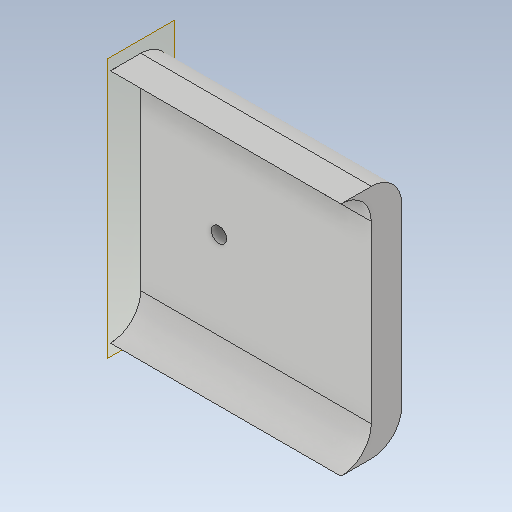
# Autodesk Inventor part: AzureKinectCradle
Saved by Autodesk Inventor 2020.2 (Build 242310000, 310)
## iProperties
Created: 2020-02-21
Part Number: AzureKinectCradle
Material: 一般
Document SubType Name: Modeling
Designer: gisen
Density: 1 g/cm^3
Appearance: 既定
Author: gisen
Autodesk Inventor part; units mm, degrees
ref_plane "YZ Plane" through (0, 0, 0) normal (1, 0, 0) x (0, 1, 0)
ref_plane "XZ Plane" through (0, 0, 0) normal (0, 1, 0) x (-1, 0, 0)
ref_plane "XY Plane" through (0, 0, 0) normal (0, 0, 1) x (1, 0, 0)
ref_plane "作業平面1" through (-27.3255, 41.0319, 38.0074) normal (1, 0, 0) x (0, 1, 0)
sketch "スケッチ2" plane through (-27.3255, 41.0319, 38.0074) normal (1, 0, 0) x (0, 1, 0)
  arc A0 (-51.6, -13.3) -> (-38.35, -26.55) centre (-38.35, -13.3) ccw
  line L0 (-51.6, 0) -> (-51.6, -13.3)
  arc A1 (-51.6, 0) -> (-38.35, -13.25) centre (-38.35, 0) ccw
  line L1 (38.35, -13.25) -> (-38.35, -13.25)
  arc A2 (38.35, -13.25) -> (51.6, 0) centre (38.35, 0) ccw
  line L2 (51.6, -13.3) -> (51.6, 0)
  arc A3 (38.35, -26.55) -> (51.6, -13.3) centre (38.35, -13.3) ccw
  line L3 (-38.35, -26.55) -> (38.35, -26.55)
  point P0 (-41.0319, -38.0074)
  constraints: 8 end point, 8 point on circle, 4 centre point
extrude "押し出し1" add sketch "スケッチ2" along normal blind 100.9
sketch "スケッチ3" plane through (-27.3255, 2.6819, 11.4574) normal (0, 0, -1) x (-1, 0, 0)
  line L0 (0, 76.7) -> (-100.9, 76.7) projected
  line L1 (-100.9, 0) -> (-100.9, 76.7) projected
  line L2 (0, 0) -> (-100.9, 0) projected
  line L3 (0, 76.7) -> (0, 0) projected
  point P0 (-27.3255, -2.6819)
  point P1 (-90.9, 66.7)
  point P2 (-90.9, 10)
  point P3 (-15, 10)
  point P4 (-15, 66.7)
  dimension "d2" = 10
  dimension "d3" = 10
  dimension "d4" = 10
  dimension "d5" = 10
  dimension "d6" = 10
  dimension "d7" = 15
  dimension "d8" = 15
  dimension "d9" = 10
  measures "d2" distance from line of L0 point (-90.9, 66.7)
  measures "d3" distance from line of L1 point (-90.9, 66.7)
  measures "d4" distance from line of L1 point (-90.9, 10)
  measures "d5" distance from line of L2 point (-90.9, 10)
  measures "d6" distance from line of L2 point (-15, 10)
  measures "d7" distance from line of L3 point (-15, 10)
  measures "d8" distance from line of L3 point (-15, 66.7)
  measures "d9" distance from line of L0 point (-15, 66.7)
hole "穴2" at (63.5745, 69.3819, 11.4574) at (63.5745, 12.6819, 11.4574) at (-12.3255, 12.6819, 11.4574) at (-12.3255, 69.3819, 11.4574) direction (0, 0, 1) diameter 3.3 depth 10.979 tip angle 118 countersink diameter 4 countersink angle 90
sketch "スケッチ4" plane through (-27.3255, 2.6819, 11.4574) normal (0, 0, -1) x (-1, 0, 0)
  circle A0 centre (-34.275, 38.35) radius 4.175 projected
  circle A1 centre (-34.275, 38.35) radius 3.35
  point P0 (-27.3255, -2.6819)
  dimension "d24" = 6.7
  constraints: 1 centre point, 1 coincident
  measures "d24" diameter of A1
hole "穴3" at (6.9495, 41.0319, 11.4574) direction (0, 0, 1) diameter 6.7 depth 15 tip angle 118 counterbore diameter 9 counterbore depth 5
